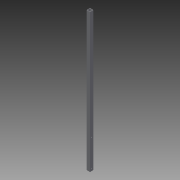
# Autodesk Inventor part: arm-vertical
Saved by Autodesk Inventor 2014 (Build 180170000, 170)
## iProperties
Created: 2014-03-22
Part Number: arm-vertical
Material: Generic
Document SubType Name: Modeling
Designer: jferner
Density: 1 g/cm^3
Appearance: Default
sqAlumWallThickness: 0.063 in
sqAlumWidth: 0.750 in
Author: jferner
Autodesk Inventor part; units mm, degrees
ref_plane "YZ Plane" through (0, 0, 0) normal (1, 0, 0) x (0, 1, 0)
ref_plane "XZ Plane" through (0, 0, 0) normal (0, 1, 0) x (-1, 0, 0)
ref_plane "XY Plane" through (0, 0, 0) normal (0, 0, 1) x (1, 0, 0)
sketch "Sketch1" plane through (0, 0, 0) normal (0, 1, 0) x (-1, 0, 0)
  line L0 (0, 0) -> (19.05, 0)
  line L1 (19.05, 0) -> (19.05, 19.05)
  line L2 (19.05, 19.05) -> (0, 19.05)
  line L3 (0, 19.05) -> (0, 0)
  line L4 (1.5875, 17.4625) -> (17.4625, 17.4625)
  line L5 (17.4625, 17.4625) -> (17.4625, 1.5875)
  line L6 (17.4625, 1.5875) -> (1.5875, 1.5875)
  line L7 (1.5875, 1.5875) -> (1.5875, 17.4625)
  dimension "d0" = 19.05
  dimension "sqAlumWidth" = 19.05
  dimension "sqAlumWallThickness" = 1.5875
  dimension "d3" = 1.5875
  dimension "d4" = 1.5875
  dimension "d5" = 1.5875
  constraints: 16 end point, 4 parallel, 2 horizontal, 2 perpendicular
  measures "d0" distance of L0.end L1.end
  measures "sqAlumWidth" distance of L1.end L2.end
  measures "sqAlumWallThickness" distance between parallel lines of L0 L6
  measures "d3" distance between parallel lines of L3 L7
  measures "d4" distance between parallel lines of L2 L4
  measures "d5" distance between parallel lines of L1 L5
extrude "Extrusion1" add sketch "Sketch1" along normal blind 765.175
sketch "Sketch2" plane through (0, 0, 19.05) normal (1, 0, 0) x (0, 0, -1)
  line L0 (0, 0) -> (19.05, 0) projected
  line L1 (19.05, 0) -> (19.05, 765.175) projected
  circle A0 centre (9.525, 12.7) radius 2.4805
  circle A1 centre (9.525, 161.925) radius 2.4805
  dimension "d8" = 4.9609
  dimension "d9" = 149.225
  dimension "screwDistanceFromBottom" = 12.7
  dimension "d11" = 9.525
  constraints: 2 centre point, 1 equal radius, 1 vertical alignment
  measures "d8" diameter of A1
  measures "d9" distance of A1.centre A0.centre
  measures "screwDistanceFromBottom" distance from line of L0 A0.centre
  measures "d11" distance from line of L1 A0.centre
extrude "Extrusion2" cut sketch "Sketch2" against normal through all
equation "\"d0\" = sqAlumWidth"
equation "\"d3\" = sqAlumWallThickness"
equation "\"d4\" = sqAlumWallThickness"
equation "\"d5\" = sqAlumWallThickness"
equation "\"d6\" = heightAboveTv + largeScrewDistance + topLargeScrewDistanceFromTop + screwDistanceFromBottom"
equation "\"d8\" = largeScrewDiameter"
equation "\"d9\" = largeScrewDistance"
equation "\"d11\" = 0.5 * sqAlumWidth"
equation "\"heightAboveTv\" = 304.8"
equation "\"largeScrewDistance\" = 149.225"
equation "\"topLargeScrewDistanceFromTop\" = 298.45"
equation "\"largeScrewDiameter\" = 4.960938"
body "Solid1"
